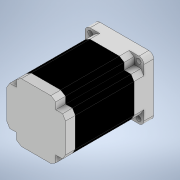
# Autodesk Inventor part: servo motor
Saved by Autodesk Inventor 2021 (Build 250183000, 183)
## iProperties
Created: 2021-06-30
Part Number: servo motor
Material: Generic
Document SubType Name: Modeling
Designer: Safiya
Density: 1 g/cm^3
Appearance: Default
Author: Safiya
Autodesk Inventor part; units mm, degrees
ref_plane "YZ Plane" through (0, 0, 0) normal (1, 0, 0) x (0, 1, 0)
ref_plane "XZ Plane" through (0, 0, 0) normal (0, 1, 0) x (-1, 0, 0)
ref_plane "XY Plane" through (0, 0, 0) normal (0, 0, 1) x (1, 0, 0)
sketch "Sketch1" plane through (0, 0, 0) normal (0, 0, 1) x (1, 0, 0)
  line L0 (-762, -762) -> (762, -762)
  line L1 (762, -762) -> (762, 762)
  line L2 (762, 762) -> (-762, 762)
  line L3 (-762, 762) -> (-762, -762)
  line L4 (-762, -762) -> (762, 762) construction
  line L5 (762, -762) -> (-762, 762) construction
  point P0 (0, 0)
  dimension "d0" = 1524
  dimension "d1" = 1524
  constraints: 12 end point, 2 midpoint, 2 parallel, 1 horizontal, 1 perpendicular
  measures "d0" distance of L2.end L1.end
  measures "d1" distance of L1.end L0.end
extrude "Extrusion1" add sketch "Sketch1" along normal blind 254
sketch "Sketch2" plane through (0, 0, 254) normal (0, 0, 1) x (1, 0, 0)
  line L0 (762, -762) -> (762, 762) projected
  line L1 (762, 762) -> (-762, 762) projected
  line L2 (-762, 762) -> (-762, -762) projected
  line L3 (-762, -762) -> (762, -762) projected
  line L4 (762, 762) -> (-762, 762) projected
  line L5 (0, 762) -> (-381, 762)
  line L6 (-381, 762) -> (-508, 685.8)
  line L7 (-508, 685.8) -> (-508, 508)
  line L8 (-508, 508) -> (-685.8, 508)
  line L9 (-685.8, 508) -> (-762, 381)
  line L10 (-762, 762) -> (-762, -762) projected
  line L11 (0, 0) -> (-762, 0)
  line L12 (0, 762) -> (0, 0)
  line L13 (381, 762) -> (508, 685.8)
  line L14 (508, 685.8) -> (508, 508)
  line L15 (508, 508) -> (685.8, 508)
  line L16 (685.8, 508) -> (762, 381)
  line L17 (0, 0) -> (762, 0)
  line L18 (0, -762) -> (-381, -762)
  line L19 (-381, -762) -> (-508, -685.8)
  line L20 (-508, -685.8) -> (-508, -508)
  line L21 (-508, -508) -> (-685.8, -508)
  line L22 (-685.8, -508) -> (-762, -381)
  line L23 (381, -762) -> (508, -685.8)
  line L24 (508, -685.8) -> (508, -508)
  line L25 (508, -508) -> (685.8, -508)
  line L26 (685.8, -508) -> (762, -381)
  dimension "d4" = 381
  dimension "d5" = 76.2
  dimension "d6" = 127
  dimension "d7" = 254
  dimension "d8" = 127
  dimension "d9" = 76.2
  constraints: 42 end point, 16 symmetric about line, 3 midpoint, 3 perpendicular, 2 point on line
  measures "d4" distance of L5.start L5.end
  measures "d5" vertical distance of L6.end L5.end
  measures "d6" horizontal distance of L5.end L6.end
  measures "d7" distance between parallel lines of L8 L1
  measures "d8" vertical distance of L8.end L9.end
  measures "d9" horizontal distance of L8.end L9.end
extrude "Extrusion2" add sketch "Sketch2" along normal blind 254 contours L26 L25 L24 L23 L3 L19 L20 L21 L22 L2 L11 L17 L0 | L17 L12 L1 L13 L14 L15 L16 L0 | L11 L2 L9 L8 L7 L6 L1 L12
sketch "Sketch3" plane through (0, 0, 508) normal (0, 0, 1) x (1, 0, 0)
  line L0 (-508, -508) -> (-508, -685.8) projected
  line L1 (-508, -685.8) -> (-381, -762) projected
  line L2 (-381, -762) -> (381, -762) projected
  line L3 (381, -762) -> (508, -685.8) projected
  line L4 (508, -685.8) -> (508, -508) projected
  line L5 (508, -508) -> (685.8, -508) projected
  line L6 (685.8, -508) -> (762, -381) projected
  line L7 (762, -381) -> (762, 381) projected
  line L8 (762, 381) -> (685.8, 508) projected
  line L9 (685.8, 508) -> (508, 508) projected
  line L10 (508, 508) -> (508, 685.8) projected
  line L11 (508, 685.8) -> (381, 762) projected
  line L12 (381, 762) -> (-381, 762) projected
  line L13 (-381, 762) -> (-508, 685.8) projected
  line L14 (-508, 685.8) -> (-508, 508) projected
  line L15 (-508, 508) -> (-685.8, 508) projected
  line L16 (-685.8, 508) -> (-762, 381) projected
  line L17 (-762, 381) -> (-762, -381) projected
  line L18 (-762, -381) -> (-685.8, -508) projected
  line L19 (-685.8, -508) -> (-508, -508) projected
  point P0 (0, 0)
extrude "Extrusion3" add sketch "Sketch3" along normal blind 1524 separate body
sketch "Sketch4" plane through (0, 0, 2032) normal (0, 0, 1) x (1, 0, 0)
  line L0 (-508, -685.8) -> (-381, -762) projected
  line L1 (-381, -762) -> (381, -762) projected
  line L2 (381, -762) -> (508, -685.8) projected
  line L3 (508, -685.8) -> (508, -508) projected
  line L4 (508, -508) -> (685.8, -508) projected
  line L5 (685.8, -508) -> (762, -381) projected
  line L6 (762, -381) -> (762, 381) projected
  line L7 (762, 381) -> (685.8, 508) projected
  line L8 (685.8, 508) -> (508, 508) projected
  line L9 (508, 508) -> (508, 685.8) projected
  line L10 (508, 685.8) -> (381, 762) projected
  line L11 (381, 762) -> (-381, 762) projected
  line L12 (-381, 762) -> (-508, 685.8) projected
  line L13 (-508, 685.8) -> (-508, 508) projected
  line L14 (-508, 508) -> (-685.8, 508) projected
  line L15 (-685.8, 508) -> (-762, 381) projected
  line L16 (-762, 381) -> (-762, -381) projected
  line L17 (-762, -381) -> (-685.8, -508) projected
  line L18 (-685.8, -508) -> (-508, -508) projected
  line L19 (-508, -508) -> (-508, -685.8) projected
  point P0 (0, 0)
extrude "Extrusion4" add sketch "Sketch4" along normal blind 254 separate body
fillet "Fillet1" radius 127 1 edges at (762, 762, 127)
fillet "Fillet2" radius 127 1 edges at (-762, 762, 127)
fillet "Fillet3" radius 127 1 edges at (762, -762, 127)
fillet "Fillet4" radius 127 1 edges at (-762, -762, 127)
sketch "Sketch5" plane through (0, 0, 0) normal (0, 0, -1) x (-1, 0, 0)
  line L0 (627.5737, -645.4476) -> (-627.5737, -645.4476) construction
  line L1 (-627.5737, -645.4476) -> (-627.5737, 645.4476) construction
  line L2 (-627.5737, 645.4476) -> (627.5737, 645.4476) construction
  line L3 (627.5737, 645.4476) -> (627.5737, -645.4476) construction
  line L4 (627.5737, -645.4476) -> (-627.5737, 645.4476) construction
  line L5 (-627.5737, -645.4476) -> (627.5737, 645.4476) construction
  point P0 (0, 0)
  constraints: 12 end point, 2 midpoint, 2 parallel, 1 horizontal, 1 perpendicular
hole "Hole1" at (-627.5737, 645.4476, 0) at (627.5737, 645.4476, 0) at (627.5737, -645.4476, 0) at (-627.5737, -645.4476, 0) direction (0, 0, 1) diameter 127 end through all bodies 1
sketch "Sketch6" plane through (0, 0, 0) normal (0, 0, -1) x (-1, 0, 0)
  circle A0 centre (0, 0) radius 508
  circle A1 centre (0, 0) radius 457.2
  dimension "d27" = 1016
  dimension "d28" = 914.4
  constraints: 2 centre point, 2 coincident
  measures "d27" diameter of A0
  measures "d28" diameter of A1
extrude "Extrusion5" cut sketch "Sketch6" against normal blind 12.7 bodies 1
sketch "Sketch7" plane through (0, 0, 0) normal (0, 0, -1) x (-1, 0, 0)
  circle A0 centre (0, 0) radius 101.6
  line L0 (-50.8, 152.4) -> (50.8, 152.4)
  line L1 (50.8, 152.4) -> (50.8, -152.4)
  line L2 (50.8, -152.4) -> (-50.8, -152.4)
  line L3 (-50.8, -152.4) -> (-50.8, 152.4)
  line L4 (-50.8, 152.4) -> (50.8, -152.4) construction
  line L5 (50.8, 152.4) -> (-50.8, -152.4) construction
  line L6 (152.4, -50.8) -> (-152.4, -50.8)
  line L7 (-152.4, -50.8) -> (-152.4, 50.8)
  line L8 (-152.4, 50.8) -> (152.4, 50.8)
  line L9 (152.4, 50.8) -> (152.4, -50.8)
  line L10 (152.4, -50.8) -> (-152.4, 50.8) construction
  line L11 (-152.4, -50.8) -> (152.4, 50.8) construction
  point P0 (-50.8, 87.9882)
  point P1 (-87.9882, 50.8)
  point P2 (-87.9882, -50.8)
  point P3 (-50.8, -87.9882)
  point P4 (50.8, -87.9882)
  point P5 (87.9882, -50.8)
  point P6 (87.9882, 50.8)
  point P7 (50.8, 87.9882)
  dimension "d31" = 203.2
  dimension "d32" = 101.6
  dimension "d33" = 304.8
  dimension "d34" = 304.8
  dimension "d35" = 101.6
  constraints: 24 end point, 4 midpoint, 4 parallel, 2 horizontal, 2 perpendicular, 1 centre point, 1 coincident
  measures "d31" diameter of A0
  measures "d32" distance of L1.end L2.end
  measures "d33" distance of L0.end L1.end
  measures "d34" distance of L6.start L6.end
  measures "d35" distance of L8.end L6.start
extrude "Extrusion6" cut sketch "Sketch7" against normal through all bodies 1
sketch "Sketch8" plane through (0, 0, 508) normal (0, 0, -1) x (-1, 0, 0)
  circle A0 centre (0, 0) radius 101.6
  dimension "d38" = 203.2
  constraints: 1 centre point, 1 coincident
  measures "d38" diameter of A0
extrude "Extrusion7" add sketch "Sketch8" along normal blind 1016 bodies 2
sketch "Sketch9" plane through (0, 0, -508) normal (0, 0, -1) x (-1, 0, 0)
  arc A0 (-87.9882, -50.8) -> (-50.8, -87.9882) centre (0, 0) ccw projected
  line L0 (-67.2021, -76.2) -> (74.5023, -76.2)
  circle A1 centre (0, 0) radius 101.6 projected
  point P0 (-50.8, -87.9882)
  point P1 (67.2021, -76.2)
  dimension "d41" = 76.2
  constraints: 2 end point, 1 horizontal, 1 point on circle
  measures "d41" distance from line of L0 point (0, 0)
extrude "Extrusion8" cut sketch "Sketch9" against normal blind 381 contours L0 A1 A0 picked at (-7.2553, -86.1155) bodies 2
sketch "Sketch10" plane through (0, 0, -508) normal (0, 0, -1) x (-1, 0, 0)
  point P0 (0, 0)
  point P1 (0, 0)
  constraints: 1 coincident
hole "Hole2" at (0, 0, -508) direction (0, 0, 1) diameter 63.5 end through all countersink diameter 127 countersink angle 82 bodies 2
sketch "Sketch11" plane through (0, 0, 0) normal (0, 0, -1) x (-1, 0, 0)
  circle A0 centre (0, 0) radius 31.75 projected
  arc A1 (355.6, 95.8829) -> (95.8829, 355.6) centre (0, 0) ccw construction
  arc A2 (404.6483, 109.1081) -> (109.1081, 404.6483) centre (0, 0) ccw
  arc A3 (306.5517, 82.6577) -> (82.6577, 306.5517) centre (0, 0) ccw
  arc A4 (306.5517, 82.6577) -> (404.6483, 109.1081) centre (355.6, 95.8829) ccw
  arc A5 (109.1081, 404.6483) -> (82.6577, 306.5517) centre (95.8829, 355.6) ccw
  dimension "d51" = 368.3
  dimension "d52" = 50.8
  dimension "d53" = 355.6
  dimension "d54" = 355.6
  constraints: 10 point on circle, 5 centre point, 4 tangent, 1 coincident
  measures "d51" radius of A1
  measures "d52" radius of A5
  measures "d53" vertical distance of A1.centre A1.end
  measures "d54" horizontal distance of A1.start A1.centre
extrude "Extrusion9" cut sketch "Sketch11" against normal blind 12.7 contours A4 A3 A5 A2 bodies 1
pattern_circular "Circular Pattern1" count 4 over 360 about axis through (0, 0, 0) along (0, 0, 1) of "Extrusion9" bodies 1
body "Solid1"
body "Solid2"
body "Solid3"
